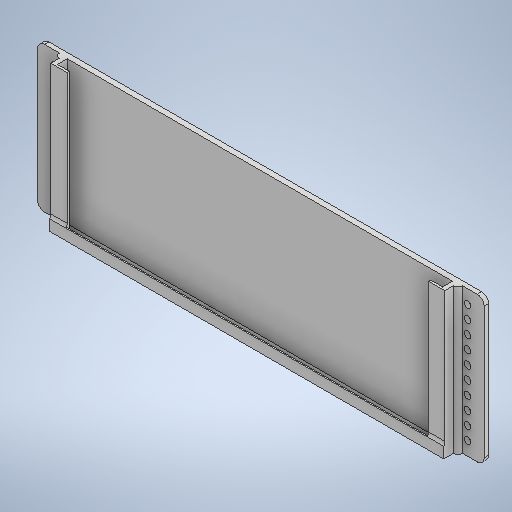
# Autodesk Inventor part: alliancePltHldr
Saved by Autodesk Inventor 2025 (Build 290162010, 162A)
## iProperties
Created: 2024-10-23
Part Number: alliancePltHldr
Material: Generic
Document SubType Name: Modeling
Designer: dcfam
Density: 1 g/cm^3
Appearance: Default
Author: dcfam
Autodesk Inventor part; units mm, degrees
ref_plane "YZ Plane" through (0, 0, 0) normal (1, 0, 0) x (0, 1, 0)
ref_plane "XZ Plane" through (0, 0, 0) normal (0, 1, 0) x (-1, 0, 0)
ref_plane "XY Plane" through (0, 0, 0) normal (0, 0, 1) x (1, 0, 0)
sketch "Sketch1" plane through (0, 0, 0) normal (0, 0, 1) x (1, 0, 0)
  line L0 (-90.25, -33.25) -> (90.25, -33.25)
  line L1 (90.25, -33.25) -> (90.25, 33.25)
  line L2 (90.25, 33.25) -> (-90.25, 33.25)
  line L3 (-90.25, 33.25) -> (-90.25, -33.25)
  line L4 (-90.25, -33.25) -> (90.25, 33.25) construction
  line L5 (90.25, -33.25) -> (-90.25, 33.25) construction
  point P0 (0, 0)
  dimension "d0" = 180.5
  dimension "d1" = 66.5
  constraints: 12 end point, 2 midpoint, 2 parallel, 1 horizontal, 1 perpendicular
  measures "d0" distance of L2.end L1.end
  measures "d1" distance of L2.end L0.start
extrude "Extrusion1" add sketch "Sketch1" along normal blind 2.5
sketch "Sketch2" plane through (0, 0, 2.5) normal (0, 0, 1) x (1, 0, 0)
  line L0 (-90.25, 33.25) -> (-90.25, -33.25) projected
  line L1 (90.25, -33.25) -> (90.25, 33.25) projected
  line L2 (-90.25, -32.25) -> (90.25, -32.25)
  line L3 (90.25, -32.25) -> (90.25, -33.25)
  line L4 (90.25, -33.25) -> (-90.25, -33.25)
  line L5 (-90.25, -33.25) -> (-90.25, -32.25)
  line L6 (-90.25, -33.25) -> (90.25, -33.25) projected
  point P0 (0, 0)
  dimension "d4" = 1
  constraints: 8 end point, 2 parallel, 2 point on line, 1 collinear, 1 horizontal, 1 perpendicular
  measures "d4" distance of L2.end L3.end
extrude "Extrusion2" add sketch "Sketch2" along normal blind 6
sketch "Sketch3" plane through (0, 0, 2.5) normal (0, 0, 1) x (1, 0, 0)
  line L0 (-90.25, -32.25) -> (90.25, -32.25) projected
  line L1 (90.25, -32.25) -> (90.25, 33.25) projected
  line L2 (90.25, 33.25) -> (-90.25, 33.25) projected
  line L3 (-90.25, 33.25) -> (-90.25, -32.25) projected
  line L4 (90.25, -33.25) -> (90.25, -32.25) projected
  line L5 (90.25, -32.25) -> (-90.25, -32.25) projected
  line L6 (-90.25, -32.25) -> (-90.25, -33.25) projected
  line L7 (-90.25, -33.25) -> (90.25, -33.25) projected
  line L8 (-90.25, 33.25) -> (-88.25, 33.25)
  line L9 (-88.25, 33.25) -> (-88.25, -32.25)
  line L10 (-88.25, -32.25) -> (-90.25, -32.25)
  line L11 (-90.25, -32.25) -> (-90.25, 33.25)
  line L12 (90.25, -32.25) -> (-90.25, -32.25) projected
  line L13 (0, 33.25) -> (0, -32.25) construction
  line L14 (-88.25, -32.25) -> (-90.25, -32.25)
  line L15 (90.25, -32.25) -> (-90.25, -32.25)
  line L16 (-90.25, 33.25) -> (90.25, 33.25)
  line L17 (90.25, 33.25) -> (90.25, -32.25)
  line L18 (-90.25, -32.25) -> (90.25, -32.25)
  line L19 (88.25, 33.25) -> (88.25, -32.25)
  line L20 (88.25, -32.25) -> (90.25, -32.25)
  point P0 (0, 0)
  dimension "d7" = 2
  constraints: 24 end point, 9 symmetric about line, 2 horizontal, 2 midpoint, 2 parallel, 1 collinear, 1 perpendicular
  measures "d7" distance of L9.end L10.end
extrude "Extrusion3" add sketch "Sketch3" along normal blind 5.5 contours L3 L2 L9 L0 | L19 L2 L1 L0
sketch "Sketch4" plane through (-88.25, -32.25, 2.5) normal (1, 0, 0) x (0, 0, -1)
  line L0 (0, 65.5) -> (0, 0) projected
  line L1 (0, 65.5) -> (-5.5, 65.5) projected
  line L2 (-5.5, 0) -> (-5.5, 65.5) projected
  line L3 (0, 0) -> (-5.5, 0) projected
  line L4 (-5.5, 65.5) -> (-4.5, 65.5)
  line L5 (-4.5, 65.5) -> (-4.5, 0)
  line L6 (-4.5, 0) -> (-5.5, 0)
  line L7 (-5.5, 0) -> (-5.5, 65.5)
  point P0 (2.5, 32.25)
  dimension "d10" = 1
  constraints: 8 end point, 2 parallel, 1 horizontal, 1 perpendicular, 1 point on line
  measures "d10" distance of L5.end L6.end
extrude "Extrusion4" add sketch "Sketch4" along normal blind 5.5 contours L5 L3 L2 L1
sketch "Sketch5" plane through (88.25, -32.25, 2.5) normal (-1, 0, 0) x (0, 0, 1)
  line L0 (0, 0) -> (0, 65.5) projected
  line L1 (5.5, 0) -> (0, 0) projected
  line L2 (5.5, 65.5) -> (5.5, 0) projected
  line L3 (0, 65.5) -> (5.5, 65.5) projected
  line L4 (5.5, 0) -> (0, 0) projected
  line L5 (5.5, 65.5) -> (4.5, 65.5)
  line L6 (4.5, 65.5) -> (4.5, 0)
  line L7 (4.5, 0) -> (5.5, 0)
  line L8 (5.5, 0) -> (5.5, 65.5)
  point P0 (-2.5, 32.25)
  dimension "d13" = 1
  constraints: 8 end point, 2 parallel, 1 horizontal, 1 perpendicular, 1 point on line
  measures "d13" distance of L7.end L6.end
extrude "Extrusion5" add sketch "Sketch5" along normal blind 5.5 contours L6 L3 L2 L1
sketch "Sketch6" plane through (-90.25, -32.25, 8.5) normal (0, 1, 0) x (1, 0, 0)
  line L0 (180.5, 0.5) -> (173, 0.5) projected
  line L1 (173, 0.5) -> (173, 1.5) projected
  line L2 (173, 1.5) -> (178.5, 1.5) projected
  line L3 (178.5, 1.5) -> (178.5, 6) projected
  line L4 (2, 6) -> (178.5, 6) projected
  line L5 (2, 6) -> (2, 1.5) projected
  line L6 (2, 1.5) -> (7.5, 1.5) projected
  line L7 (7.5, 1.5) -> (7.5, 0.5) projected
  line L8 (7.5, 0.5) -> (0, 0.5) projected
  line L9 (0, 0.5) -> (0, 0) projected
  line L10 (180.5, 0) -> (0, 0) projected
  line L11 (180.5, 0.5) -> (180.5, 0) projected
  line L12 (180.5, 0.5) -> (0, 0.5)
  line L13 (0, 0.5) -> (0, 0)
  line L14 (0, 0) -> (180.5, 0)
  line L15 (180.5, 0) -> (180.5, 0.5)
  point P0 (90.25, 8.5)
  constraints: 8 end point, 2 parallel, 1 horizontal, 1 perpendicular
extrude "Extrusion6" add sketch "Sketch6" along normal blind 4 contours L11 L10 L9 L8 L12 L0
fillet "Fillet1" radius 3.175 2 edges at (86.5, -28.25, 8) (-86.5, -28.25, 8)
sketch "Sketch7" plane through (0, 0, 0) normal (0, 0, 1) x (1, 0, 0)
  line L0 (-82.75, -26.5397) -> (-90.25, -26.5397) projected
  line L1 (-82.75, 33.25) -> (-82.75, -26.5397) projected
  line L2 (-90.25, 33.25) -> (-82.75, 33.25) projected
  line L3 (-90.25, 33.25) -> (-90.25, -26.5397) projected
  line L4 (90.25, -33.25) -> (90.25, -28.25) projected
  line L5 (82.75, -28.25) -> (90.25, -28.25) projected
  line L6 (-82.75, -28.25) -> (82.75, -28.25) projected
  line L7 (-90.25, -28.25) -> (-82.75, -28.25) projected
  line L8 (-90.25, -33.25) -> (-90.25, -28.25) projected
  line L9 (-90.25, -33.25) -> (90.25, -33.25) projected
  line L10 (-82.75, -26.5397) -> (-90.25, -26.5397) projected
  line L11 (-90.25, 33.25) -> (-99.075, 33.25)
  line L12 (-102.25, 30.075) -> (-102.25, -30.075)
  line L13 (-99.075, -33.25) -> (-90.25, -33.25)
  line L14 (-90.25, -33.25) -> (-90.25, 33.25)
  arc A0 (-99.075, 33.25) -> (-102.25, 30.075) centre (-99.075, 30.075) ccw
  arc A1 (-102.25, -30.075) -> (-99.075, -33.25) centre (-99.075, -30.075) ccw
  line L15 (-88.25, 33.25) -> (-88.25, -32.25) projected
  line L16 (-88.25, -32.25) -> (88.25, -32.25) projected
  line L17 (88.25, -32.25) -> (88.25, 33.25) projected
  line L18 (88.25, 33.25) -> (-88.25, 33.25) projected
  line L19 (0, 33.25) -> (0, -33.25) construction
  line L20 (90.25, 33.25) -> (99.075, 33.25)
  line L21 (102.25, 30.075) -> (102.25, -30.075)
  line L22 (99.075, -33.25) -> (90.25, -33.25)
  arc A2 (102.25, 30.075) -> (99.075, 33.25) centre (99.075, 30.075) ccw
  arc A3 (99.075, -33.25) -> (102.25, -30.075) centre (99.075, -30.075) ccw
  line L23 (-90.25, 33.25) -> (-90.25, -33.25)
  line L24 (90.25, 33.25) -> (90.25, -33.25)
  point P0 (0, 0)
  point P1 (-102.25, -33.25)
  dimension "d19" = 12
  dimension "d20" = 3.175
  constraints: 20 end point, 8 point on circle, 8 symmetric about line, 4 centre point, 4 tangent, 3 parallel, 2 midpoint, 2 point on line, 1 equal radius, 1 horizontal, 1 perpendicular, 1 vertical, 2 other
  measures "d19" distance of L13.end point (-102.25, -33.25)
  measures "d20" radius of A0
extrude "Extrusion7" add sketch "Sketch7" along normal blind 2 contours L14 L8 L13 A1 L12 A0 L11 L3 | L24 L20 A2 L21 A3 L22 L4
sketch "Sketch8" plane through (0, 0, 2) normal (0, 0, 1) x (1, 0, 0)
  line L0 (-90.25, 33.25) -> (-99.075, 33.25) construction
  line L1 (-94.6625, 33.25) -> (-94.6625, -33.25) construction
  line L2 (-99.075, -33.25) -> (-90.25, -33.25) construction
  line L3 (88.25, 33.25) -> (-88.25, 33.25) construction
  line L4 (0, 33.25) -> (0, -33.25) construction
  line L5 (-90.25, -33.25) -> (90.25, -33.25) construction
  circle A0 centre (-94.6625, 27) radius 1.5
  circle A1 centre (-94.6625, 21) radius 1.5
  circle A2 centre (-94.6625, 15) radius 1.5
  circle A3 centre (-94.6625, 9) radius 1.5
  circle A4 centre (-94.6625, 3) radius 1.5
  circle A5 centre (-94.6625, -3) radius 1.5
  circle A6 centre (-94.6625, -9) radius 1.5
  circle A7 centre (-94.6625, -15) radius 1.5
  circle A8 centre (-94.6625, -21) radius 1.5
  circle A9 centre (-94.6625, -27) radius 1.5
  line L6 (-94.6625, 3) -> (-94.6625, -3) construction
  line L7 (-94.6625, -3) -> (-94.6625, 0) construction
  line L8 (-94.6625, 3) -> (-94.6625, -3) construction
  line L9 (-94.6625, 0) -> (-102.084, 0) construction
  line L10 (-102.25, 30.075) -> (-102.25, -30.075) construction
  line L11 (-102.25, 0) -> (-90.25, 0) construction
  circle A10 centre (94.6625, 27) radius 1.5
  circle A11 centre (94.6625, 21) radius 1.5
  circle A12 centre (94.6625, 15) radius 1.5
  circle A13 centre (94.6625, 9) radius 1.5
  circle A14 centre (94.6625, 3) radius 1.5
  circle A15 centre (94.6625, -3) radius 1.5
  circle A16 centre (94.6625, -9) radius 1.5
  circle A17 centre (94.6625, -15) radius 1.5
  circle A18 centre (94.6625, -21) radius 1.5
  circle A19 centre (94.6625, -27) radius 1.5
  point P0 (0, 0)
  dimension "d23" = 3
  dimension "d26" = 6
  constraints: 20 centre point, 14 end point, 10 symmetric about line, 6 midpoint, 3 vertical, 2 horizontal, 1 collinear, 1 point on line, 28 other
  measures "d23" diameter of A0
  measures "d26" distance of A0.centre A1.centre
extrude "Extrusion8" cut sketch "Sketch8" against normal blind 546
fillet "Fillet2" radius 2.032 2 edges at (90.25, 0, 2) (-90.25, 0, 2) inverted yes
body "Solid1"
